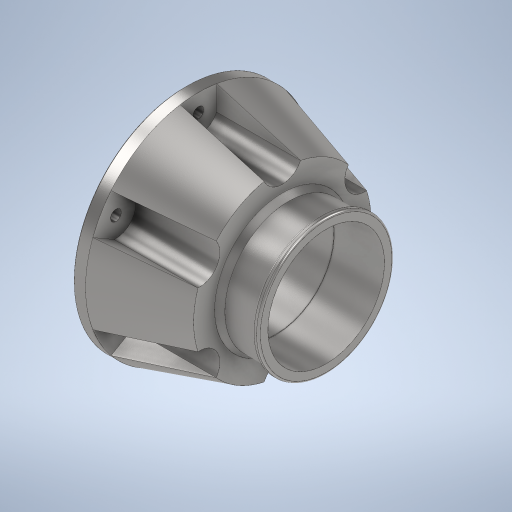
# Autodesk Inventor part: bauteil_externe
Saved by Autodesk Inventor 2024 (Build 280153000, 153)
## iProperties
Created: 2024-02-01
Part Number: bauteil_externe
Material: Stahl, galvanisiert
Document SubType Name: Modeling
Designer: ffogue
Density: 7.85 g/cm^3
Appearance: Galvanisiert
Author: ffogue
Autodesk Inventor part; units mm, degrees
ref_plane "YZ Plane" through (0, 0, 0) normal (1, 0, 0) x (0, 1, 0)
ref_plane "XZ Plane" through (0, 0, 0) normal (0, 1, 0) x (-1, 0, 0)
ref_plane "XY Plane" through (0, 0, 0) normal (0, 0, 1) x (1, 0, 0)
sketch "Skizze1" plane through (0, 0, 0) normal (0, 0, 1) x (1, 0, 0)
  line L0 (-56, 0) -> (-56, 90)
  line L1 (-56, 90) -> (-46, 90)
  line L2 (-46, 90) -> (21, 70.7881)
  line L3 (21, 70.7881) -> (21, 51)
  line L4 (21, 51) -> (51, 51)
  line L5 (51, 51) -> (51, 54)
  line L6 (51, 54) -> (56, 54)
  line L7 (56, 54) -> (56, 0)
  line L8 (-56, 0) -> (56, 0)
  point P0 (0, 0)
  point P1 (53.5, 54)
  point P2 (0, 0)
  dimension "d0" = 112
  dimension "d1" = 16
  dimension "d2" = 108
  dimension "d3" = 180
  dimension "d4" = 102
  dimension "d5" = 77
  dimension "d6" = 10
  dimension "d7" = 5
  constraints: 18 end point, 4 perpendicular, 2 midpoint, 2 parallel, 1 coincident, 1 horizontal, 1 vertical
  measures "d0" distance of L0.start L7.end
  measures "d1" angle of L2 L1
  measures "d2" diameter of point (53.5, 54) L8
  measures "d3" diameter of L1 L8
  measures "d4" diameter of L4 L8
  measures "d5" distance from line of L3 L0.end
  measures "d6" distance from line of L1.end L0
  measures "d7" distance between parallel lines of L7 L5
revolve "Umdrehung1" add sketch "Skizze1" angle 360 about axis through (-56, 0, 0) along (1, 0, 0)
fillet "Rundung1" radius 1.2 1 edges at (51, -51, 0)
fillet "Rundung2" radius 1.5 1 edges at (51, -54, 0)
fillet "Rundung3" radius 1.5 1 edges at (56, -54, 0)
sketch "Skizze2" plane through (21, 0, 0) normal (1, 0, 0) x (0, 0, -1)
  circle A0 centre (0, 0) radius 90 projected
  line L0 (126, 0) -> (-126, 0) projected
  circle A1 centre (0, 0) radius 90 projected
  circle A2 centre (0, 0) radius 70.7881 projected
  arc A3 (-69.2826, -14.5216) -> (-69.2826, 14.5216) centre (-76, 0) ccw
  line L1 (-88.8207, 14.5216) -> (-69.2826, 14.5216)
  line L2 (-69.2826, -14.5216) -> (-88.8207, -14.5216)
  point P0 (0, 0)
  point P1 (-79.0517, 14.5216)
  point P2 (-79.0517, 14.5216)
  dimension "d16" = 16
  dimension "d54" = 76
  constraints: 6 point on circle, 4 end point, 1 centre point, 1 coincident, 1 horizontal, 1 midpoint, 1 parallel, 1 point on line
  measures "d16" radius of A3
  measures "d54" distance of point (0, 0) A3.centre
extrude "Extrusion3" cut sketch "Skizze2" against normal blind 67 contours L1 A2 L0 A0 | A0 L0 A2 L2 | A3 L0 A2 | A2 L0 A3 picked at (-76.7377, 8.0985) picked at (-76.7377, -8.0985) picked at (-67.2736, 2.8267) picked at (-67.2736, -2.8267)
sketch "Skizze9" plane through (-46, 0, 0) normal (1, 0, 0) x (0, 0, -1)
  arc A0 (-69.2826, -14.5216) -> (-69.2826, 14.5216) centre (-76, 0) ccw projected
  point P0 (0, 0)
  constraints: 1 coincident
hole "Bohrung3" at (-46, 0, 76) direction (-1, 0, 0) diameter 8.5 end through all
pattern_circular "Runde Anordnung1" count 6 over 360 about axis through (-12.5, 0, 0) along (1, 0, 0) of "Extrusion3", "Bohrung3"
chamfer "Fasen1" distance 1 angle 45 1 edges at (-56, -90, 0)
chamfer "Fasen3" distance 3 angle 60 1 edges at (21, -51, 0) measured on face at (21, 19.1412, 59.8068)
sketch "Skizze11" plane through (-56, 0, 0) normal (-1, 0, 0) x (0, 0, 1)
  circle A0 centre (0, 0) radius 90 projected
  point P0 (0, 0)
  point P1 (0, 0)
  constraints: 1 coincident
hole "Bohrung4" at (-56, 0, 0) direction (1, 0, 0) diameter 92 depth 79 counterbore diameter 98 counterbore depth 7
sketch "Skizze12" plane through (56, 0, 0) normal (1, 0, 0) x (0, 0, -1)
  circle A0 centre (0, 0) radius 54 projected
  point P0 (0, 0)
  constraints: 1 coincident
hole "Bohrung5" at (56, 0, 0) direction (-1, 0, 0) diameter 93 depth 40
chamfer "Fasen4" distance 1 angle 60 1 edges at (-56, 0, -49) measured on face at (-56, 18.4136, -67.5369)
chamfer "Fasen5" distance 1.6 angle 60 1 edges at (-49, 0, -46) measured on face at (-49, 0, -46.8427)
fillet "Rundung6" radius 0.4 1 edges at (-49, 0, -49)
